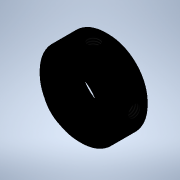
# Autodesk Inventor part: SCBRJ10-13_b
Saved by Autodesk Inventor 2021 (Build 250183000, 183)
## iProperties
Created: 2025-01-05
Part Number: SCBRJ10-13_b
Material: Generic
Catalog Web Link: www.cadenas.de
Description: SCBRJ, PSCBRJ, SSCBRJ, SCSRAJ, SCSRAWJ, SCBSJ, PSCBSJ, SSCBSJ_body-Set Collars - For Bearing Fixing - (For Space Saving) - Set Screw Compact Type
Vendor: MISUMI
Document SubType Name: Modeling
Designer: psAdmin
Manufacturer: MISUMI
Mass: 0.911864 g
Surface Area: 8.85581 cm^2
Volume: 0.911864 cm^3
Density: 1 g/cm^3
Appearance: PSOLRGB-0-0-0
Category: PARTsolutions
Company: MISUMI
Title: SCBRJ10-13
Author: Cadenas PARTsolutions
Comments: Set Collars - For Bearing Fixing - (For Space Saving) - Set Screw Compact Type
PSOL_IDENT_0: {$CADENAS_DATA/23d-libs/misumi/metric/03_set_collars/scbrj/scbrj_b.prj},238 {VTYP=3D},{NB=SCBRJ10-13
PSOL_IDENT_1: _b},{LINA=SCBRJ10-13},{NN=SCBRJ, PSCBRJ, SSCBRJ, SCSRAJ, SCSRAWJ, SCBSJ, PSCBSJ, SSCBSJ_body},{DATE=
PSOL_IDENT_2: 02.11.2021 00:56:13},{GEOMDATE=19.10.2021 09:28:48},{VERSION=},{LINEID=60},{WBVAR=TS,MAT,ST,DSS},{WB
PSOL_IDENT_3: NUMERIC=DSS}  {NB=SCBRJ10-13_b},{LINA=SCBRJ10-13},{KT=DUMMY},{PN=SCBRJ10-13},{D=10},{TYPE=SCBRJ},{TS=
PSOL_IDENT_4: SN},{MAT=1045},{MATA='1045','1045 Carbon Steel','304','SUS304 Equivalent','2017','2017 Aluminum Allo
PSOL_IDENT_5: y'},{ST=Black Oxide},{AC=Set Screws 2 Pcs.},{DSS=13},{DS1=13,14,16},{AB=6800ZZ(19)},{B11=7.5},{B12=1
PSOL_IDENT_6: 0},{D1=17},{M=M3x3},{THMD=3},{THDMIN=2.459},{BB=6},{ST0='Black Oxide','Black Oxide','Electroless Nic
PSOL_IDENT_7: kel Plating','Electroless Nickel Plating'},{C=0.5},{L=3},{TS1='SN','Short Nose','LN','Long Nose'},{C
PSOL_IDENT_8: OLOR=0.00,0.00,0.00,0.00},{B=7.5},{B1=0},{LTHREAD=3}
NB: SCBRJ10-13_b
NN: SCBRJ, PSCBRJ, SSCBRJ, SCSRAJ, SCSRAWJ, SCBSJ, PSCBSJ, SSCBSJ_body
NT: Set Collars - For Bearing Fixing - (For Space Saving) - Set Screw Compact Type
NBSYN: $PN._b
LINA: SCBRJ10-13
CATALOG: Misumi
PN: SCBRJ10-13
D: 10
TS: Short Nose
MAT: 1045 Carbon Steel
ST: Black Oxide
DSS: 13
D1: 17
M: M3x3
BB: 6
C: 0.5
L: 3
B: 7.5
B1: 0
SUPPLIER: MISUMI
ARTICLENO: SCBRJ10-13_b
BOMINFO: SCBRJ10-13
CREATOR: CADENAS GmbH
Autodesk Inventor part; units mm, degrees
sketch "Sketch_1" plane through (0, 0, 0) normal (0, 1, 0) x (-1, 0, 0)
  line L0 (0, 4.5) -> (0, -3)
  line L1 (-5, 4) -> (-5.5, 4.5)
  line L2 (-5.5, 4.5) -> (-6, 4.5)
  line L3 (-6, 4.5) -> (-6.5, 4)
  line L4 (-6.5, 4) -> (-6.5, 3)
  line L5 (-6.5, 3) -> (-8, 3)
  line L6 (-8, 3) -> (-8.5, 2.5)
  line L7 (-8.5, 2.5) -> (-8.5, -2.5)
  line L8 (-8.5, -2.5) -> (-8, -3)
  line L9 (-8, -3) -> (-5.5, -3)
  line L10 (-5.5, -3) -> (-5, -2.5)
  line L11 (-5, -2.5) -> (-5, 4)
  constraints: 24 end point
revolve "Revolution1" add sketch "Sketch_1" angle 360 about axis through (0, 0, 4.5) along (0, 0, -1)
sketch "Sketch_8" plane through (0, 0, 0) normal (0, 0, 1) x (1, 0, 0)
  line L0 (8.5, 0) -> (4, 0)
  line L1 (4, 0) -> (4, 1.2295)
  line L2 (4, 1.2295) -> (8.2295, 1.2295)
  line L3 (8.2295, 1.2295) -> (8.5, 1.5)
  line L4 (8.5, 1.5) -> (8.5, 0)
  line L5 (8.5, 0) -> (4, 0)
  constraints: 12 end point
revolve "Revolution2" cut sketch "Sketch_8" angle 360 about axis through (8.5, 0, 0) along (-1, 0, 0)
thread "Thread1" size "M3x0.5" class "6H" standard "ISO Metric profile" full length
sketch "Sketch_2" plane through (0, 0, 0) normal (0, 0, 1) x (1, 0, 0)
  line L0 (0, 8.5) -> (0, 4)
  line L1 (0, 4) -> (-1.2295, 4)
  line L2 (-1.2295, 4) -> (-1.2295, 8.2295)
  line L3 (-1.2295, 8.2295) -> (-1.5, 8.5)
  line L4 (-1.5, 8.5) -> (0, 8.5)
  line L5 (0, 8.5) -> (0, 4)
  constraints: 12 end point
revolve "Revolution3" cut sketch "Sketch_2" angle 360 about axis through (0, 8.5, 0) along (0, -1, 0)
thread "Thread2" size "M3x0.5" class "6H" standard "ISO Metric profile" full length
ref_plane "body_set_h_XY" through (0, 8.5, 0) normal (0, 1, 0) x (1, 0, 0)
ref_plane "body_set_h_YZ" through (0, 8.5, 0) normal (1, 0, 0) x (0, 0, -1)
ref_plane "body_set_h_ZX" through (0, 8.5, 0) normal (0, 0, -1) x (0, 1, 0)
ref_plane "body_set_v_XY" through (8.5, 0, 0) normal (1, 0, 0) x (0, 0, -1)
ref_plane "body_set_v_YZ" through (8.5, 0, 0) normal (0, 0, -1) x (0, 1, 0)
ref_plane "body_set_v_ZX" through (8.5, 0, 0) normal (0, 1, 0) x (1, 0, 0)
body "Solid1"
